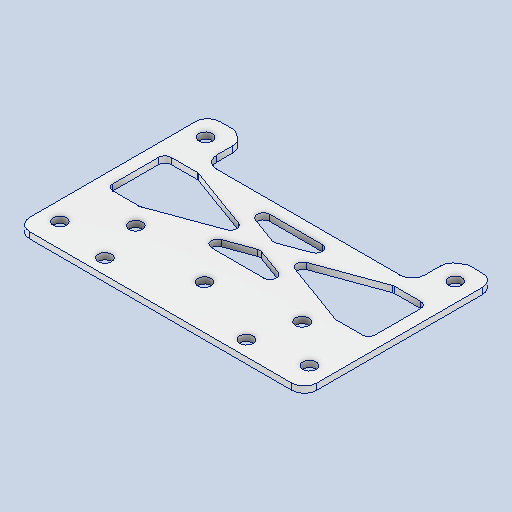
# Autodesk Inventor part: upper_plate_under
Saved by Autodesk Inventor 2024.1 (Build 281209000, 209)
## iProperties
Created: 2025-02-03
Part Number: upper_plate_under
Material: アルミニウム 6061
Document SubType Name: Sheet Metal
Designer: hibik
Density: 2.7 g/cm^3
Sheet Metal Rule: Default_mm
Appearance: アルミニウム - フラット
Author: hibik
Autodesk Inventor part; units mm, degrees
ref_plane "YZ Plane" through (0, 0, 0) normal (1, 0, 0) x (0, 1, 0)
ref_plane "XZ Plane" through (0, 0, 0) normal (0, 1, 0) x (-1, 0, 0)
ref_plane "XY Plane" through (0, 0, 0) normal (0, 0, 1) x (1, 0, 0)
sketch "スケッチ1" plane through (0, 0, 0) normal (0, 1, 0) x (-1, 0, 0)
  line L0 (75, 0) -> (105, -51.9615)
  line L1 (-75, 0) -> (-105, -51.9615)
  line L2 (0, -218.2384) -> (0, 36.3731)
  line L3 (147, 0) -> (-147, 0)
  line L4 (105, -51.9615) -> (30, -181.8653)
  line L5 (30, -181.8653) -> (-30, -181.8653)
  line L6 (-30, -181.8653) -> (-105, -51.9615)
  line L7 (75, 0) -> (-75, 0)
  line L8 (34, 0) -> (34, -24.3509)
  line L9 (34, -24.3509) -> (48.7058, -49.822)
  line L10 (48.7058, -49.822) -> (90, -25.9808)
  line L11 (45, 0) -> (45, -18) construction
  line L12 (45, -18) -> (34, -24.3509) construction
  line L13 (84.5, -87.4686) -> (63.4115, -75.2931)
  line L14 (63.4115, -75.2931) -> (48.7058, -49.822)
  line L15 (-34, 0) -> (-34, -24.3509)
  line L16 (-34, -24.3509) -> (-48.7058, -49.822)
  line L17 (-63.4115, -75.2931) -> (-48.7058, -49.822)
  line L18 (-84.5, -87.4686) -> (-63.4115, -75.2931)
  circle A0 centre (30, -32.75) radius 1.6
  circle A1 centre (-30, -32.75) radius 1.6
  line L19 (35.5295, -27) -> (-35.5295, -27)
  point P0 (0, 0)
  point P1 (0, 0)
  point P2 (0, -27)
  dimension "d1" = 150
  dimension "d2" = 60
  dimension "d3" = 60
  dimension "d6" = 60
  dimension "d30" = 60
  dimension "d31" = 18
  dimension "d32" = 30
  dimension "d33" = 41
  dimension "d34" = 3.2
  dimension "d35" = 30
  dimension "d36" = 32.75
  dimension "d37" = 27
  measures "d1" distance of L1.start L0.start
  measures "d2" angle of L3 L0
  measures "d3" angle of L1 L3
  measures "d6" distance of L4.end L5.end
  measures "d30" angle of L11 L12
  measures "d31" distance of L11.start L11.end
  measures "d32" distance of L0.start L11.start
  measures "d33" distance of L0.start L8.start
  measures "d34" diameter of A0
  measures "d35" distance from line of L2 A0.centre
  measures "d36" distance from line of L7 A0.centre
  measures "d37" distance between parallel lines of L7 L19
extrude "プレート1" add sketch "スケッチ1" along normal blind 1.5 contours L14 L13 L4 L5 L2 L19 L9 | L2 L5 L6 L18 L17 L16 L19
sketch "スケッチ4" plane through (0, 1.5, 0) normal (0, 1, 0) x (1, 0, 0)
  circle A0 centre (30, 67.8013) radius 1.6
  circle A1 centre (45, 67.8013) radius 1.6
  line L0 (0, 218.2384) -> (0, -36.3731)
  circle A2 centre (-30, 67.8013) radius 1.6
  circle A3 centre (-45, 67.8013) radius 1.6
  line L1 (61.6173, 73.1025) -> (25, 73.1025) construction
  line L2 (25, 73.1025) -> (25, 62.5) construction
  line L3 (-61.6173, 73.1025) -> (-25, 73.1025) construction
  line L4 (-25, 73.1025) -> (-25, 62.5) construction
  line L5 (-25, 62.5) -> (25, 62.5)
  line L6 (30, 73.1025) -> (30, 181.8653)
  line L7 (30, 181.8653) -> (-30, 181.8653)
  line L8 (-30, 181.8653) -> (-30, 73.1025)
  line L9 (-25, 62.5) -> (25, 62.5)
  line L10 (25, 62.5) -> (25, 71.0141)
  line L11 (-25, 71.0141) -> (-25, 62.5)
  line L12 (30, 181.8653) -> (84.5, 87.4686)
  line L13 (76.75, 100.892) -> (30, 73.9008)
  line L14 (-30, 73.9008) -> (-76.75, 100.892)
  line L15 (-84.5, 87.4686) -> (-30, 181.8653)
  line L16 (84.5, 87.4686) -> (63.4115, 75.2931)
  line L17 (-63.4115, 75.2931) -> (-84.5, 87.4686)
  line L18 (-35.5295, 27) -> (-63.4115, 75.2931)
  line L19 (62.8673, 70.9375) -> (54.6673, 85.1403)
  arc A4 (54.6673, 85.1403) -> (44.275, 79.1403) centre (49.4712, 82.1403) ccw
  line L20 (44.275, 79.1403) -> (52.475, 64.9375)
  line L21 (52.475, 64.9375) -> (62.8673, 70.9375)
  line L22 (51.2321, 85.1903) -> (52.993, 82.1403)
  line L23 (52.993, 82.1403) -> (51.2321, 79.0903)
  line L24 (51.2321, 79.0903) -> (47.7102, 79.0903)
  line L25 (47.7102, 79.0903) -> (45.9493, 82.1403)
  line L26 (45.9493, 82.1403) -> (47.7102, 85.1903)
  line L27 (47.7102, 85.1903) -> (51.2321, 85.1903)
  line L28 (-30, 73.9008) -> (-25, 71.0141)
  line L29 (30, 73.9008) -> (25, 71.0141)
  point P0 (0, 0)
extrude "切り取り3" cut sketch "スケッチ4" against normal blind 1.5 contours A0 | A1 | L7 L6 L29 L10 L5 L0 | L0 L5 L11 L28 L8 L7 | L12 L13 A4 L6 | L8 L14 L15 | A4 L13 L27 L26 | L26 L27 L13 | A2 | A3
sketch "スケッチ5" plane through (0, 1.5, 0) normal (0, 1, 0) x (1, 0, 0)
  line L0 (-75, 44) -> (75, 44) projected
  circle A0 centre (-20, 41) radius 3
  circle A1 centre (20, 41) radius 3
  line L1 (-25, 62.5) -> (25, 62.5) projected
  line L2 (0, 62.5) -> (0, 27)
  line L3 (35.5295, 27) -> (-35.5295, 27) projected
  circle A2 centre (-20, 41) radius 1.6
  circle A3 centre (20, 41) radius 1.6
  circle A4 centre (0, 37.5) radius 1.6
  point P0 (0, 0)
  dimension "d41" = 6
  dimension "d42" = 6
  dimension "d43" = 40
  dimension "d44" = 3.2
  dimension "d45" = 3.2
  dimension "d46" = 3.2
  dimension "d47" = 3.5
  constraints: 5 centre point, 2 coincident, 2 end point, 2 midpoint, 1 point on line, 1 symmetric about line, 1 tangent
  measures "d41" diameter of A0
  measures "d42" diameter of A1
  measures "d43" distance of A1.centre A0.centre
  measures "d44" diameter of A2
  measures "d45" diameter of A3
  measures "d46" diameter of A4
  measures "d47" vertical distance of A0.centre A4.centre
extrude "切り取り4" cut sketch "スケッチ5" against normal blind 1.5 contours A4 L2 | L2 A4 | A2 | A3
sketch "スケッチ6" plane through (0, 1.5, 0) normal (0, 1, 0) x (1, 0, 0)
  ellipse E0 centre (-73.3666, 93.1522) end of major axis (-72.2841, 92.5272) minor radius 1.2133 projected
  circle A0 centre (-48.4391, 79.9279) radius 1.6
  circle A1 centre (-73.3666, 93.1522) radius 1.6
  line L0 (0, 0) -> (0, 20.4537)
  circle A2 centre (48.4391, 79.9279) radius 1.6
  circle A3 centre (73.3666, 93.1522) radius 1.6
  circle A4 centre (-48.4391, 79.9279) radius 1.35 projected
  dimension "d51" = 3.2
  dimension "d52" = 3.2
  constraints: 4 centre point, 2 end point, 2 symmetric about line, 1 coincident, 1 vertical, 2 other
  measures "d51" diameter of A0
  measures "d52" diameter of A1
extrude "切り取り5" cut sketch "スケッチ6" against normal blind 1.5 contours E0 | A0 | A1 | A2 | A3 | A4
fillet "フィレット2" radius 3 12 edges at (-84.5, 0.75, -87.4686) (-76.75, 0.75, -100.892) (-63.4115, 0.75, -75.2931) (-35.5295, 0.75, -27) (35.5295, 0.75, -27) (63.4115, 0.75, -75.2931) (84.5, 0.75, -87.4686) (76.75, 0.75, -100.892) (25, 0.75, -62.5) (-25, 0.75, -62.5) (-25, 0.75, -71.0141) (25, 0.75, -71.0141)
sketch "スケッチ7" plane through (0, 1.5, 0) normal (0, 1, 0) x (1, 0, 0)
  line L0 (-34.5, 72.8013) -> (34.5, 72.8013)
  line L1 (34.5, 72.8013) -> (34.5, 27)
  line L2 (34.5, 27) -> (-34.5, 27)
  line L3 (-34.5, 27) -> (-34.5, 72.8013)
  line L4 (33.7974, 27) -> (-33.7974, 27) projected
  circle A0 centre (30, 32.75) radius 1.6 projected
  circle A1 centre (30, 67.8013) radius 1.6 projected
  arc A2 (26.5, 71.8801) -> (25, 69.282) centre (28, 69.282) ccw projected
  line L5 (25, 69.282) -> (25, 65.5) projected
  arc A3 (22, 62.5) -> (25, 65.5) centre (22, 65.5) ccw projected
  line L6 (22, 62.5) -> (-22, 62.5) projected
  arc A4 (-25, 65.5) -> (-22, 62.5) centre (-22, 65.5) ccw projected
  line L7 (-25, 65.5) -> (-25, 69.282) projected
  arc A5 (-25, 69.282) -> (-26.5, 71.8801) centre (-28, 69.282) ccw projected
  line L8 (-26.5, 71.8801) -> (-74.1519, 99.392) projected
  arc A6 (-74.1519, 99.392) -> (-78.25, 98.2939) centre (-75.6519, 96.7939) ccw projected
  line L9 (-83, 90.0666) -> (-78.25, 98.2939) projected
  arc A7 (-83, 90.0666) -> (-81.9019, 85.9686) centre (-80.4019, 88.5666) ccw projected
  line L10 (-64.1077, 75.6951) -> (-81.9019, 85.9686) projected
  arc A8 (-63.0096, 74.597) -> (-64.1077, 75.6951) centre (-65.6077, 73.097) ccw projected
  line L11 (-36.3955, 28.5) -> (-63.0096, 74.597) projected
  arc A9 (-36.3955, 28.5) -> (-33.7974, 27) centre (-33.7974, 30) ccw projected
  line L12 (33.7974, 27) -> (-33.7974, 27) projected
  arc A10 (33.7974, 27) -> (36.3955, 28.5) centre (33.7974, 30) ccw projected
  line L13 (63.0096, 74.597) -> (36.3955, 28.5) projected
  arc A11 (64.1077, 75.6951) -> (63.0096, 74.597) centre (65.6077, 73.097) ccw projected
  line L14 (81.9019, 85.9686) -> (64.1077, 75.6951) projected
  arc A12 (81.9019, 85.9686) -> (83, 90.0666) centre (80.4019, 88.5666) ccw projected
  line L15 (78.25, 98.2939) -> (83, 90.0666) projected
  arc A13 (78.25, 98.2939) -> (74.1519, 99.392) centre (75.6519, 96.7939) ccw projected
  line L16 (74.1519, 99.392) -> (26.5, 71.8801) projected
  circle A14 centre (48.4391, 79.9279) radius 1.6 projected
  circle A15 centre (-48.4391, 79.9279) radius 1.6 projected
  circle A16 centre (-73.3666, 93.1522) radius 1.6 projected
  circle A17 centre (73.3666, 93.1522) radius 1.6 projected
  circle A18 centre (-20, 41) radius 1.6 projected
  circle A19 centre (0, 37.5) radius 1.6 projected
  circle A20 centre (20, 41) radius 1.6 projected
  circle A21 centre (-30, 32.75) radius 1.6 projected
  circle A22 centre (30, 32.75) radius 1.6 projected
  circle A23 centre (-45, 67.8013) radius 1.6 projected
  circle A24 centre (45, 67.8013) radius 1.6 projected
  circle A25 centre (30, 67.8013) radius 1.6 projected
  circle A26 centre (-30, 67.8013) radius 1.6 projected
  point P0 (0, 0)
  point P1 (0, 27)
  point P2 (26.3711, 71.8013)
  point P3 (33.5, 27)
  point P4 (-33.7974, 27)
  point P5 (-33.5, 27)
  point P6 (-26.3711, 71.8013)
  point P7 (-28.0955, 72.8013)
  point P8 (-34.5, 27.0834)
  point P9 (34.5, 27.0834)
  point P10 (28.0955, 72.8013)
  dimension "d56" = 4.5
  dimension "d57" = 5
  constraints: 8 end point, 2 midpoint, 2 parallel, 1 collinear, 1 horizontal, 1 perpendicular
  measures "d56" distance from line of L1 A0.centre
  measures "d57" distance from line of L0 A1.centre
extrude "押し出し1" cut sketch "スケッチ7" against normal through all contours L3 A9 L11 A8 L10 A7 L9 A6 L8 L0 | L16 A13 L15 A12 L14 A11 L13 A10 L1 L0 | A14 | A15 | A16 | A17 | A23 | A24
fillet "フィレット3" radius 3 4 edges at (34.5, 0.75, -72.8013) (-34.5, 0.75, -72.8013) (34.5, 0.75, -27.0834) (-34.5, 0.75, -27.0834)
sketch "スケッチ8" plane through (0, 1.5, 0) normal (0, 1, 0) x (1, 0, 0)
  circle A0 centre (-17, 30.5787) radius 1.6 projected
  circle A1 centre (17, 30.5787) radius 1.6 projected
  point P0 (0, 0)
extrude "切り取り6" cut sketch "スケッチ8" against normal blind 1.5
sketch "スケッチ9" plane through (0, 1.5, 0) normal (0, 1, 0) x (1, 0, 0)
  line L0 (-31.5, 59.5) -> (31.5, 59.5)
  line L1 (31.5, 59.5) -> (31.5, 45.5)
  line L2 (31.5, 45.5) -> (-31.5, 45.5)
  line L3 (-31.5, 45.5) -> (-31.5, 59.5)
  line L4 (-18.136, 45.5) -> (-14.636, 42)
  line L5 (-14.636, 42) -> (14.636, 42)
  line L6 (14.636, 42) -> (18.136, 45.5)
  line L7 (0, 87.3615) -> (0, -14.5603) projected
  line L8 (22, 62.5) -> (-22, 62.5) projected
  line L9 (-34.5, 69.8013) -> (-34.5, 30) projected
  circle A0 centre (0, 37.5) radius 1.6 projected
  circle A1 centre (20, 41) radius 1.6 projected
  line L10 (-14.7681, 59.5) -> (0, 54.0972)
  line L11 (14.7681, 59.5) -> (0, 54.0972)
  line L12 (-23.5, 59.5) -> (-4.3659, 52.5)
  line L13 (-4.3659, 52.5) -> (-23.5, 45.5)
  line L14 (-14.7681, 45.5) -> (0, 50.9028)
  line L15 (0, 50.9028) -> (14.7681, 45.5)
  line L16 (23.5, 45.5) -> (4.3659, 52.5)
  line L17 (4.3659, 52.5) -> (23.5, 59.5)
  line L18 (-14.7681, 45.5) -> (-17.234, 44.5979)
  line L19 (14.7681, 45.5) -> (17.234, 44.5979)
  line L20 (-14.636, 42) -> (-14.636, 36)
  line L21 (-14.636, 36) -> (-11.636, 33)
  line L22 (-11.636, 33) -> (-6.636, 33)
  line L23 (-6.636, 33) -> (-6.636, 42)
  line L24 (6.636, 42) -> (6.636, 33)
  line L25 (6.636, 33) -> (11.636, 33)
  line L26 (11.636, 33) -> (14.636, 36)
  line L27 (14.636, 36) -> (14.636, 42)
  point P0 (0, 0)
  point P1 (31.5, 52.5)
  dimension "d63" = 3
  dimension "d64" = 3
  dimension "d65" = 4.5
  dimension "d66" = 4.5
  dimension "d67" = 4.5
  dimension "d68" = 3
  dimension "d69" = 8
  dimension "d72" = 9
  dimension "d73" = 5
  dimension "d74" = 8
  constraints: 50 end point, 21 point on line, 5 parallel, 5 perpendicular, 4 collinear, 3 vertical, 2 horizontal, 2 vertical alignment, 1 horizontal alignment, 1 midpoint, 9 other
  measures "d63" distance between parallel lines of L8 L0
  measures "d64" distance between parallel lines of L9 L3
  measures "d65" distance from line of A0.centre L5
  measures "d66" distance from line of A1.centre L6
  measures "d67" distance from line of A1.centre L2
  measures "d68" distance between parallel lines of L10 L12
  measures "d69" distance from line of L3 L12.start
  measures "d72" distance of L24.start L24.end
  measures "d73" distance of L24.end L25.end
  measures "d74" distance between parallel lines of L27 L24
extrude "切り取り7" cut sketch "スケッチ9" against normal blind 1.5 contours L0 L12 L13 L2 L3 | L0 L7 L10 | L0 L11 L7 | L15 L2 L7 | L7 L2 L14 | L0 L1 L2 L16 L17
fillet "フィレット4" radius 1.5 16 edges at (14.7681, 0.75, -59.5) (-14.7681, 0.75, -59.5) (0, 0.75, -54.0972) (0, 0.75, -50.9028) (-14.7681, 0.75, -45.5) (14.7681, 0.75, -45.5) (-4.3659, 0.75, -52.5) (4.3659, 0.75, -52.5) (-31.5, 0.75, -59.5) (-23.5, 0.75, -59.5) (23.5, 0.75, -59.5) (31.5, 0.75, -59.5) (31.5, 0.75, -45.5) (23.5, 0.75, -45.5) (-23.5, 0.75, -45.5) (-31.5, 0.75, -45.5)
equation "\"d3\" = d2"
equation "\"d38\" = Thickness"
equation "\"d41\" = d42"
equation "\"d48\" = Thickness"
equation "\"d53\" = Thickness"
equation "\"d61\" = Thickness"
equation "\"d64\" = d63"
equation "\"d66\" = d65"
equation "\"d67\" = d65"
equation "\"d68\" = d63"
equation "\"d70\" = Thickness"
equation "\"d16\" = Thickness"
equation "\"Thickness\" = 1.5"
